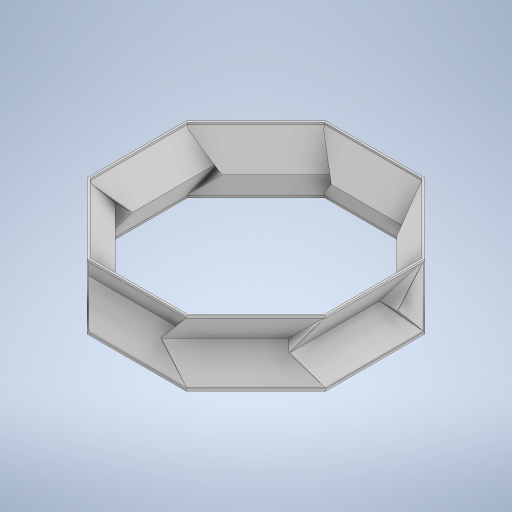
# Autodesk Inventor part: 팔각형 OV-PAM 층 한개
Saved by Autodesk Inventor 2024 (Build 280153000, 153)
## iProperties
Created: 2023-06-16
Part Number: 팔각형 OV-PAM 층 한개
Material: 일반
Document SubType Name: Modeling
Designer: jsw
Density: 1 g/cm^3
Appearance: 기본값
Author: jsw
Autodesk Inventor part; units mm, degrees
ref_plane "YZ Plane" through (0, 0, 0) normal (1, 0, 0) x (0, 1, 0)
ref_plane "XZ Plane" through (0, 0, 0) normal (0, 1, 0) x (-1, 0, 0)
ref_plane "XY Plane" through (0, 0, 0) normal (0, 0, 1) x (1, 0, 0)
sketch "스케치1" plane through (0, 0, 0) normal (0, 1, 0) x (-1, 0, 0)
  line L0 (-46.091883, 19.091883) -> (-19.091883, 46.091883)
  line L1 (-19.091883, 46.091883) -> (19.091883, 46.091883)
  line L2 (19.091883, 46.091883) -> (46.091883, 19.091883)
  line L3 (46.091883, 19.091883) -> (46.091883, -19.091883)
  line L4 (46.091883, -19.091883) -> (19.091883, -46.091883)
  line L5 (19.091883, -46.091883) -> (-19.091883, -46.091883)
  line L6 (-19.091883, -46.091883) -> (-46.091883, -19.091883)
  line L7 (-46.091883, -19.091883) -> (-46.091883, 19.091883)
  line L8 (-19.257569, 46.491883) -> (19.257569, 46.491883)
  line L9 (19.257569, 46.491883) -> (46.491883, 19.257569)
  line L10 (46.491883, 19.257569) -> (46.491883, -19.257569)
  line L11 (46.491883, -19.257569) -> (19.257569, -46.491883)
  line L12 (19.257569, -46.491883) -> (-19.257569, -46.491883)
  line L13 (-19.257569, -46.491883) -> (-46.491883, -19.257569)
  line L14 (-46.491883, -19.257569) -> (-46.491883, 19.257569)
  line L15 (-46.491883, 19.257569) -> (-19.257569, 46.491883)
  point P0 (0, 0)
  point P1 (0, 0)
  point P2 (0, 0)
  dimension "d0" = 38.18377
  dimension "d2" = 0.4
  constraints: 32 end point, 2 coincident, 2 horizontal, 34 other
  measures "d0" distance of L0.end L1.end
  measures "d2" distance between parallel lines of L10 L3
extrude "돌출2" add sketch "스케치1" along normal blind 12 contours L0 L1 L2 L3 L4 L5 L6 L7 | L8 L9 L10 L11 L12 L13 L14 L15
ref_plane "작업 평면2" through (46.491883, 0, 19.257569) normal (-0.8660254, -0.5, 0) x (0, 0, -1)
sketch "스케치3" plane through (46.491883, 0, 19.257569) normal (1, 0, 0) x (0, 0, -1)
  line L0 (0, 0) -> (0, 12)
  line L1 (0, 12) -> (38.515137, 12)
  line L2 (0, 0) -> (38.515137, 0)
  line L3 (38.515137, 0) -> (38.515137, 12)
  line L4 (38.515137, 12) -> (0, 12)
  line L5 (0, 12) -> (0, 0)
  line L6 (0, 12) -> (-7.304723, 12)
  line L7 (-27.234315, 12) -> (0, 12)
  line L8 (0, 0) -> (-7.304723, 12)
  line L9 (38.515137, 12) -> (19.257569, 12)
  line L10 (28.257569, 12) -> (38.515137, 0)
  point P0 (19.257569, 0)
  dimension "d17" = 121.33
  dimension "d49" = 9
  constraints: 16 end point, 5 midpoint, 2 parallel, 2 point on line, 1 horizontal, 1 perpendicular
  measures "d17" angle of L8 L2
  measures "d49" distance of point (19.258, 12) L10.start
extrude "돌출4" cut sketch "스케치3" against normal up to surface contours L8 L6 L0 | L0 L1 L10 L2 surface through (46.491883, 0, 19.257569) normal (-0.8660254, -0.5, 0)
pattern_circular "원형 패턴1" count 8 over 360 about axis through (0, -10, 0) along (0, 1, 0) of "돌출4"
mirror "미러5" about plane through (0, 12, 0) normal (0, 1, 0) of "돌출2", "돌출4", "원형 패턴1"
sketch "스케치9" plane through (-19.257569, 24, -46.491883) normal (0, 1, 0) x (1, 0, 0)
  line L0 (65.749452, -65.749452) -> (65.749452, -27.234315)
  line L1 (65.749452, -27.234315) -> (38.515137, 0)
  line L2 (38.515137, 0) -> (0, 0)
  line L3 (0, 0) -> (-27.234315, -27.234315)
  line L4 (-27.234315, -27.234315) -> (-27.234315, -65.749452)
  line L5 (-27.234315, -65.749452) -> (0, -92.983766)
  line L6 (0, -92.983766) -> (38.515137, -92.983766)
  line L7 (38.515137, -92.983766) -> (65.749452, -65.749452)
  point P0 (19.257569, -46.491883)
extrude "돌출8" add sketch "스케치9" along normal blind 0.8
sketch "스케치10" plane through (0, 0, 0) normal (0, -1, 0) x (1, 0, 0)
  line L0 (46.491883, 19.257569) -> (46.491883, -19.257569)
  line L1 (19.257569, 46.491883) -> (46.491883, 19.257569)
  line L2 (-19.257569, 46.491883) -> (19.257569, 46.491883)
  line L3 (-46.491883, 19.257569) -> (-19.257569, 46.491883)
  line L4 (-46.491883, -19.257569) -> (-46.491883, 19.257569)
  line L5 (-19.257569, -46.491883) -> (-46.491883, -19.257569)
  line L6 (19.257569, -46.491883) -> (-19.257569, -46.491883)
  line L7 (46.491883, -19.257569) -> (19.257569, -46.491883)
  point P0 (0, 0)
extrude "돌출9" add sketch "스케치10" along normal blind 0.8
shell "쉘6" thickness 0.4 removed faces 2 at (15.497294, 24.8, -6.41919) at (-2.658915, -0.8, 6.41919)
sketch "스케치12" plane through (-19.257569, 24.8, -46.491883) normal (0, 1, 0) x (1, 0, 0)
  line L0 (-0.165685, 0.4) -> (38.680822, 0.4)
  line L1 (38.680822, 0.4) -> (66.149452, -27.068629)
  line L2 (66.149452, -27.068629) -> (66.149452, -65.915137)
  line L3 (66.149452, -65.915137) -> (38.680822, -93.383766)
  line L4 (38.680822, -93.383766) -> (-0.165685, -93.383766)
  line L5 (-0.165685, -93.383766) -> (-27.634315, -65.915137)
  line L6 (-27.634315, -65.915137) -> (-27.634315, -27.068629)
  line L7 (-27.634315, -27.068629) -> (-0.165685, 0.4)
  line L8 (65.749452, -65.749452) -> (65.749452, -27.234315)
  line L9 (0, -92.983766) -> (38.515137, -92.983766)
  line L10 (38.349452, -92.583766) -> (0.165685, -92.583766)
  line L11 (65.349452, -27.4) -> (65.349452, -65.583766)
  line L12 (65.349452, -65.583766) -> (38.349452, -92.583766)
  line L13 (38.349452, -92.583766) -> (0.165685, -92.583766)
  line L14 (0.165685, -92.583766) -> (-26.834315, -65.583766)
  line L15 (-26.834315, -65.583766) -> (-26.834315, -27.4)
  line L16 (-26.834315, -27.4) -> (0.165685, -0.4)
  line L17 (0.165685, -0.4) -> (38.349452, -0.4)
  line L18 (38.349452, -0.4) -> (65.349452, -27.4)
  line L19 (65.749452, -27.234315) -> (38.515137, 0)
  line L20 (38.515137, 0) -> (0, 0)
  line L21 (0, 0) -> (-27.234315, -27.234315)
  line L22 (-27.234315, -27.234315) -> (-27.234315, -65.749452)
  line L23 (-27.234315, -65.749452) -> (0, -92.983766)
  line L24 (0, -92.983766) -> (38.515137, -92.983766)
  line L25 (38.515137, -92.983766) -> (65.749452, -65.749452)
  line L26 (65.749452, -65.749452) -> (65.749452, -27.234315)
  point P0 (19.257569, -46.491883)
  point P1 (19.257569, -46.491883)
  point P2 (65.749452, -27.234315)
  dimension "d50" = 0.4
  constraints: 16 end point, 1 coincident, 1 horizontal, 17 other
  measures "d50" distance between parallel lines of L8 L2
extrude "돌출10" add sketch "스케치12" against normal blind 0.8 contours L0 L1 L2 L3 L4 L5 L6 L7
ref_plane "작업 평면6" through (-19.257569, 12, -46.491883) normal (0, 1, 0) x (1, 0, 0)
mirror "미러8" about plane through (-19.257569, 12, -46.491883) normal (0, 1, 0) of "돌출10"
